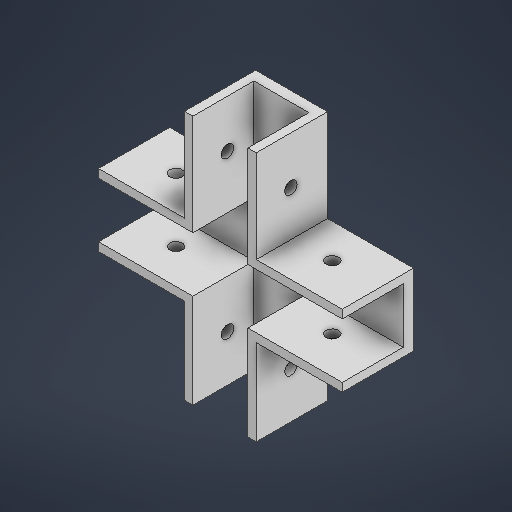
# Autodesk Inventor part: Lifter Connecter
Saved by Autodesk Inventor 2026.1 (Build 301233020, 233B)
## iProperties
Created: 2025-11-25
Part Number: Lifter Connecter
Material: Generic
Document SubType Name: Modeling
Designer: sarab
Density: 1 g/cm^3
Appearance: Default
Author: sarab
Autodesk Inventor part; units mm, degrees
ref_plane "YZ Plane" through (0, 0, 0) normal (1, 0, 0) x (0, 1, 0)
ref_plane "XZ Plane" through (0, 0, 0) normal (0, 1, 0) x (-1, 0, 0)
ref_plane "XY Plane" through (0, 0, 0) normal (0, 0, 1) x (1, 0, 0)
sketch "Sketch1" plane through (0, 0, 0) normal (0, 0, 1) x (1, 0, 0)
  line L0 (16.224, -2.484) -> (16.224, 25.338)
  line L1 (16.224, 25.338) -> (44.046, 25.338)
  line L2 (44.046, 41.562) -> (16.224, 41.562)
  line L3 (0, 41.562) -> (-27.822, 41.562)
  line L4 (-27.822, 25.338) -> (0, 25.338)
  line L5 (16.224, -2.484) -> (18.708, -2.484)
  line L6 (18.708, 44.046) -> (44.046, 44.046)
  line L7 (44.046, 22.854) -> (18.708, 22.854)
  line L8 (18.708, 22.854) -> (18.708, 0)
  line L9 (-2.484, 44.046) -> (-27.822, 44.046)
  line L10 (-27.822, 22.854) -> (-2.484, 22.854)
  line L11 (0, 0) -> (0, 25.338)
  line L12 (0, 41.562) -> (0, 71.322)
  line L13 (16.224, 71.322) -> (16.224, 41.562)
  line L14 (16.224, 25.338) -> (16.224, 0)
  line L15 (18.708, -2.484) -> (18.708, 22.854)
  line L16 (18.708, 44.046) -> (18.708, 71.322)
  line L17 (-2.484, 71.322) -> (-2.484, 44.046)
  line L18 (-2.484, 22.854) -> (-2.484, -2.484)
  line L19 (-27.822, 44.046) -> (-27.822, 41.562)
  line L20 (-27.822, 25.338) -> (-27.822, 22.854)
  line L21 (44.046, 44.046) -> (44.046, 41.562)
  line L22 (44.046, 25.338) -> (44.046, 22.854)
  line L23 (18.708, 71.322) -> (16.224, 71.322)
  line L24 (0, 71.322) -> (-2.484, 71.322)
  line L25 (-2.484, -2.484) -> (0, -2.484)
  line L26 (0, -2.484) -> (0, 1.997)
  point P0 (-25.338, 41.562)
  point P1 (-25.338, 25.338)
  constraints: 54 end point, 18 perpendicular, 8 point on line, 2 vertical, 1 horizontal
extrude "Extrusion1" add sketch "Sketch1" along normal blind 18
sketch "Sketch2" plane through (0, 0, 0) normal (0, 0, -1) x (-1, 0, 0)
  line L0 (2.484, 22.854) -> (2.484, -2.484) projected
  line L1 (27.822, 22.854) -> (2.484, 22.854) projected
  line L2 (27.822, 44.046) -> (27.822, 22.854) projected
  line L3 (2.484, 44.046) -> (27.822, 44.046) projected
  line L4 (2.484, 71.322) -> (2.484, 44.046) projected
  line L5 (-18.708, 71.322) -> (2.484, 71.322) projected
  line L6 (-18.708, 44.046) -> (-18.708, 71.322) projected
  line L7 (-44.046, 44.046) -> (-18.708, 44.046) projected
  line L8 (-44.046, 22.854) -> (-44.046, 44.046) projected
  line L9 (-18.708, 22.854) -> (-44.046, 22.854) projected
  line L10 (-18.708, -2.484) -> (-18.708, 22.854) projected
  line L11 (2.484, -2.484) -> (-18.708, -2.484) projected
  point P0 (0, 0)
extrude "Extrusion2" add sketch "Sketch2" along normal blind 3
sketch "Sketch3" plane through (-27.822, 44.046, 18) normal (0, 1, 0) x (1, 0, 0)
  circle A0 centre (12.6484, 10.1922) radius 1.841
  point P0 (27.822, 18)
  constraints: 1 centre point
extrude "Extrusion3" cut sketch "Sketch3" against normal blind 28
sketch "Sketch4" plane through (18.708, 44.046, 18) normal (0, 1, 0) x (1, 0, 0)
  circle A0 centre (11.4919, 10.9288) radius 1.841
  point P0 (-18.708, 18)
  constraints: 1 centre point
extrude "Extrusion4" cut sketch "Sketch4" against normal blind 28
sketch "Sketch5" plane through (18.708, 44.046, 18) normal (1, 0, 0) x (0, 0, -1)
  circle A0 centre (10.1922, -32.8499) radius 1.841
  circle A1 centre (10.1922, 13.2601) radius 1.841
  point P0 (18, -44.046)
  constraints: 2 centre point
extrude "Extrusion5" cut sketch "Sketch5" against normal blind 28
body "Solid1"
